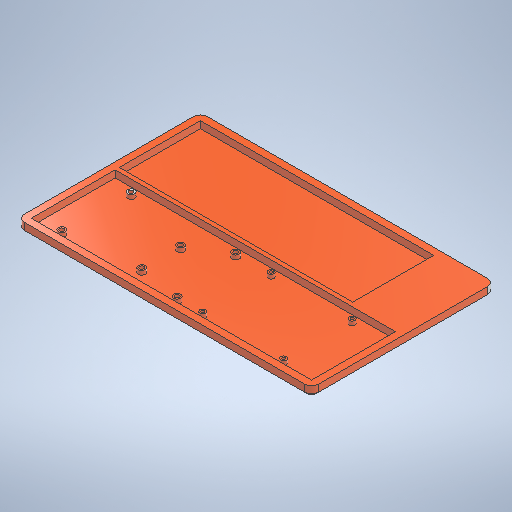
# Autodesk Inventor part: Electronic Base
Saved by Autodesk Inventor 2025.2 (Build 292293000, 293)
## iProperties
Created: 2025-02-05
Part Number: Electronic Base
Material: Generic
Document SubType Name: Modeling
Designer: caomi
Density: 1 g/cm^3
Appearance: Default
Author: caomi
Autodesk Inventor part; units mm, degrees
ref_plane "YZ Plane" through (0, 0, 0) normal (1, 0, 0) x (0, 1, 0)
ref_plane "XZ Plane" through (0, 0, 0) normal (0, 1, 0) x (-1, 0, 0)
ref_plane "XY Plane" through (0, 0, 0) normal (0, 0, 1) x (1, 0, 0)
sketch "Sketch1" plane through (0, 0, 0) normal (0, 1, 0) x (-1, 0, 0)
  line L0 (210.6, 131) -> (0, 131)
  line L1 (0, 131) -> (0, 0)
  line L2 (0, 0) -> (210.6, 0)
  line L3 (210.6, 0) -> (210.6, 131)
  line L4 (92, 68) -> (7, 68) construction
  line L5 (7, 68) -> (7, 124) construction
  line L6 (7, 124) -> (92, 124) construction
  line L7 (92, 124) -> (92, 68) construction
  circle A0 centre (88.5, 71.5) radius 1.1
  circle A1 centre (88.5, 120.5) radius 1.1
  circle A2 centre (30.5, 71.5) radius 1.1
  circle A3 centre (30.5, 120.5) radius 1.1
  line L8 (0, 0) -> (-136.9444, 0) construction
  line L9 (0, 0) -> (0, -49.9102) construction
  circle A4 centre (88.5, 71.5) radius 2.1
  circle A5 centre (88.5, 120.5) radius 2.1
  circle A6 centre (30.5, 71.5) radius 2.1
  circle A7 centre (30.5, 120.5) radius 2.1
  line L10 (205.6, 66) -> (5, 66)
  line L11 (5, 66) -> (5, 126)
  line L12 (5, 126) -> (205.6, 126)
  line L13 (205.6, 126) -> (205.6, 66)
  line L14 (203.6, 69.33) -> (102, 69.33) construction
  line L15 (102, 69.33) -> (102, 122.67) construction
  line L16 (102, 122.67) -> (203.6, 122.67) construction
  line L17 (203.6, 122.67) -> (203.6, 69.33) construction
  line L18 (205.6, 5) -> (38.6, 5)
  line L19 (38.6, 5) -> (38.6, 63)
  line L20 (38.6, 63) -> (205.6, 63)
  line L21 (205.6, 63) -> (205.6, 5)
  circle A8 centre (188.36, 71.87) radius 2.55
  circle A9 centre (188.36, 71.87) radius 1.55
  circle A10 centre (113.43, 71.87) radius 2.55
  circle A11 centre (113.43, 71.87) radius 1.55
  circle A12 centre (189.63, 120.13) radius 1.55
  circle A13 centre (107.08, 120.13) radius 2.55
  circle A14 centre (189.63, 120.13) radius 2.55
  circle A15 centre (107.08, 120.13) radius 1.55
  circle A16 centre (137.56, 115.05) radius 2.55
  circle A17 centre (137.56, 115.05) radius 1.55
  circle A18 centre (137.56, 87.11) radius 2.55
  circle A19 centre (137.56, 87.11) radius 1.55
  point P0 (92, 96)
  point P1 (102, 96)
  point P2 (1.5544, 63)
  point P3 (2.0056, 63)
  point P4 (82.8344, 63)
  point P5 (83.2856, 63)
  dimension "d8" = 85
  dimension "d9" = 56
  dimension "d10" = 2.2
  dimension "d11" = 3.5
  dimension "d12" = 3.5
  dimension "d13" = 3.5
  dimension "d33" = 1
  dimension "d34" = 1
  dimension "d35" = 1
  dimension "d36" = 1
  dimension "d44" = 58
  dimension "d48" = 53.34
  dimension "d49" = 101.6
  dimension "d50" = 167
  dimension "d51" = 58
  dimension "d52" = 5
  dimension "d55" = 2
  dimension "d56" = 2
  dimension "d57" = 2
  dimension "d58" = 10
  dimension "d59" = 5
  dimension "d60" = 15.24
  dimension "d61" = 2.54
  dimension "d62" = 3.1
  dimension "d63" = 1
  dimension "d64" = 90.17
  dimension "d65" = 13.97
  dimension "d66" = 96.52
  dimension "d68" = 66.04
  dimension "d70" = 45.72
  dimension "d71" = 17.78
  dimension "d73" = 5
  dimension "d74" = 50.8
  dimension "d76" = 3
  dimension "d77" = 2
  dimension "d78" = 5
  constraints: 44 end point, 20 centre point, 13 equal radius, 10 parallel, 6 coincident, 6 horizontal, 5 horizontal alignment, 5 perpendicular, 3 vertical alignment, 2 midpoint, 1 collinear, 1 vertical
  measures "d8" distance of L5.end L6.end
  measures "d9" distance of L4.end L5.end
  measures "d10" diameter of A0
  measures "d11" distance from line of L4 A0.centre
  measures "d12" distance from line of A0.centre L7
  measures "d13" distance from line of L6 A1.centre
  measures "d33" radial gap between concentric circles of A0 A4
  measures "d34" radial gap between concentric circles of A1 A5
  measures "d35" radial gap between concentric circles of A2 A6
  measures "d36" radial gap between concentric circles of A3 A7
  measures "d44" distance of A0.centre A2.centre
  measures "d48" distance of L16.end L14.start
  measures "d49" distance of L15.end L16.end
  measures "d50" distance of L18.start L18.end
  measures "d51" distance of L18.end L19.end
  measures "d52" distance between parallel lines of L2 L18
  measures "d55" distance between parallel lines of L11 L5
  measures "d56" distance between parallel lines of L12 L6
  measures "d57" distance between parallel lines of L17 L13
  measures "d58" distance between parallel lines of L7 L15
  measures "d59" distance between parallel lines of L13 L3
  measures "d60" distance from line of L17 A9.centre
  measures "d61" distance from line of L14 A8.centre
  measures "d62" diameter of A9
  measures "d63" radial gap between concentric circles of A8 A9
  measures "d64" distance from line of L17 A10.centre
  measures "d65" distance from line of L17 A12.centre
  measures "d66" distance from line of L17 A13.centre
  measures "d68" distance from line of L17 A16.centre
  measures "d70" distance from line of L14 A16.centre
  measures "d71" distance from line of L14 A18.centre
  measures "d73" distance between parallel lines of L0 L12
  measures "d74" distance from line of L14 A12.centre
  measures "d76" distance between parallel lines of L10 L20
  measures "d77" distance between parallel lines of L10 L4
  measures "d78" distance between parallel lines of L1 L11
extrude "Extrusion1" add sketch "Sketch1" against normal blind 2 contours L3 L2 L1 L0 | A0 | A1 | A2 | A3 | A4 | A5 | A6 | A7 | L10 L11 L12 L13 | L18 L19 L20 L21 | A8 | A9 | A10 | A11 | A12 | A13 | A14 | A15 | A16 | A17 | A18 | A19
extrude "Extrusion2" add sketch "Sketch1" along normal blind 5 contours L3 L2 L1 L0
extrude "Extrusion3" add sketch "Sketch1" along normal blind 3 contours A4 | A5 | A6 | A7 | A8 | A10 | A13 | A14 | A16 | A18
fillet "Fillet1" radius 5 4 edges at (-210.6, 1.5, 0) (0, 1.5, 131) (-210.6, 1.5, 131) (0, 1.5, 0)
chamfer "Chamfer1" distance 2 angle 45 8 edges at (-105.3, -2, 131) (-209.1355, -2, 129.5355) (-210.6, -2, 65.5) (-209.1355, -2, 1.4645) (-105.3, -2, 0) (-1.4645, -2, 1.4645) (0, -2, 65.5) (-1.4645, -2, 129.5355)
equation "\"d12\" = d11"
equation "\"d13\" = d11"
equation "\"board_border\" = 2"
equation "\"base_wall\" = 5"
body "Solid1"
